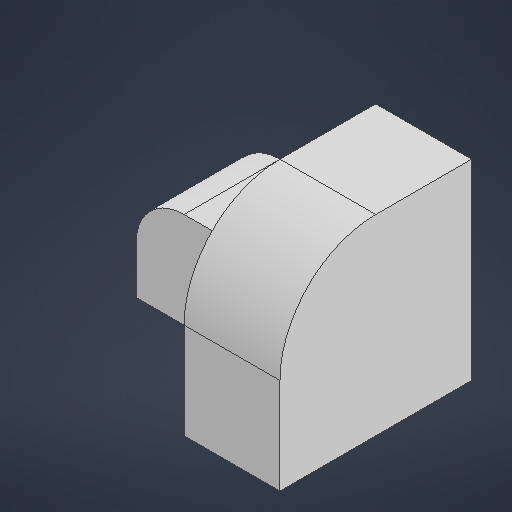
# Autodesk Inventor part: 3
Saved by Autodesk Inventor 2025.4 (Build 294407000, 407)
## iProperties
Created: 2026-05-07
Part Number: 3
Material: Generic
Document SubType Name: Modeling
Designer: VuQuan
Density: 1 g/cm^3
Appearance: Default
Author: VuQuan
Autodesk Inventor part; units mm, degrees
ref_plane "YZ Plane" through (0, 0, 0) normal (1, 0, 0) x (0, 1, 0)
ref_plane "XZ Plane" through (0, 0, 0) normal (0, 1, 0) x (-1, 0, 0)
ref_plane "XY Plane" through (0, 0, 0) normal (0, 0, 1) x (1, 0, 0)
sketch "Sketch1" plane through (0, 0, 0) normal (0, 0, 1) x (1, 0, 0)
  line L0 (0, 0) -> (50, 0)
  line L1 (50, 0) -> (50, 40)
  line L2 (50, 40) -> (30, 40)
  line L3 (30, 40) -> (30, 0)
  line L4 (0, 0) -> (0, 10)
  arc A0 (10, 20) -> (0, 10) centre (10, 10) ccw
  line L5 (10, 20) -> (20, 20)
  arc A1 (20, 20) -> (30, 30) centre (20, 30) ccw
  dimension "d0" = 50
  dimension "d1" = 40
  dimension "d2" = 20
  dimension "d3" = 20
  dimension "d4" = 10
  constraints: 12 end point, 4 perpendicular, 4 point on circle, 4 tangent, 2 centre point, 2 point on line, 1 equal radius, 1 horizontal, 1 vertical
  measures "d0" distance of L0.start L0.end
  measures "d1" distance of L0.end L1.end
  measures "d2" distance of L1.end L2.end
  measures "d3" distance between parallel lines of L0 L5
  measures "d4" radius of A1
extrude "Extrusion1" add sketch "Sketch1" along normal blind 20 contours L4 A0 L5 A1 L3 L0
extrude "Extrusion2" add sketch "Sketch1" along normal blind 40 contours L3 L2 L1 L0
fillet "Fillet1" radius 20 1 edges at (40, 40, 40)
body "Solid1"
